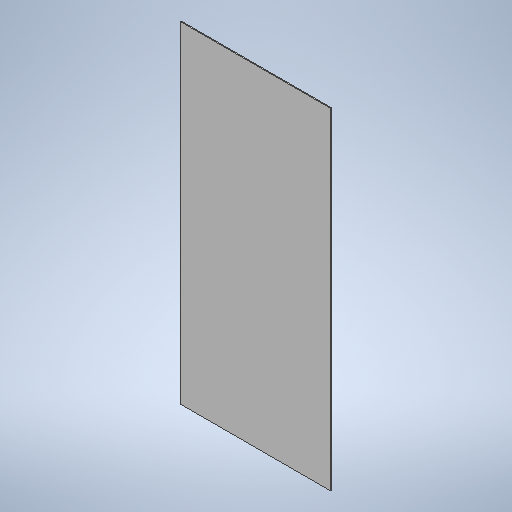
# Autodesk Inventor part: Деталь1
Saved by Autodesk Inventor 2026.2 (Build 302298000, 298)
## iProperties
Created: 2026-09-15
Part Number: Деталь1
Material: Generic
Document SubType Name: Sheet Metal
Designer: user
Density: 1 g/cm^3
Sheet Metal Rule: Default_mm
Appearance: Default
Mass: 1650 g
Surface Area: 11096 cm^2
Volume: 1650 cm^3
Flat Pattern Width: 50 cm
Flat Pattern Length: 110 cm
Flat Pattern Area: 5500 cm^2
Sheet Metal Width: 500,000 mm
Sheet Metal Length: 1100,000 mm
Sheet Metal Area: 550000,000 mm^2
Author: user
Autodesk Inventor part; units mm, degrees
ref_plane "YZ Plane" through (0, 0, 0) normal (1, 0, 0) x (0, 1, 0)
ref_plane "XZ Plane" through (0, 0, 0) normal (0, 1, 0) x (-1, 0, 0)
ref_plane "XY Plane" through (0, 0, 0) normal (0, 0, 1) x (1, 0, 0)
sketch "Эскиз1" plane through (0, 0, 0) normal (0, 0, 1) x (1, 0, 0)
  line L0 (-250, -550) -> (250, -550)
  line L1 (250, -550) -> (250, 550)
  line L2 (250, 550) -> (-250, 550)
  line L3 (-250, 550) -> (-250, -550)
  line L4 (-250, -550) -> (250, 550) construction
  line L5 (250, -550) -> (-250, 550) construction
  point P0 (0, 0)
  dimension "d0" = 500
  dimension "d1" = 1100
  measures "d0" distance of L2.end L1.end
  measures "d1" distance of L1.end L0.end
extrude "Пластина1" add sketch "Эскиз1" along normal blind 3
equation "\"d2\" = Толщина"
equation "\"Радиус_гибки\" = Толщина"
equation "\"Ширина_просечки\" = Толщина"
equation "\"Глубина_просечки\" = 0.5 * Толщина"
equation "\"Размер_просечки\" = 4 * Толщина"
equation "\"Мин_остаток\" = 2 * Толщина"
equation "\"Радиус_перехода\" = Радиус_гибки"
equation "\"Радиус_Якоби\" = Радиус_гибки"
equation "\"Размер_зазора\" = Толщина"
equation "\"Толщина\" = 3"
